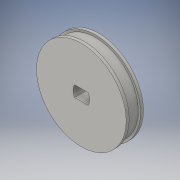
# Autodesk Inventor part: big tire sumo robot
Saved by Autodesk Inventor 2016 (Build 200138000, 138)
## iProperties
Created: 2017-09-06
Part Number: big tire sumo robot
Material: Generic
Document SubType Name: Modeling
Designer: student
Density: 1 g/cm^3
Appearance: Default
Author: student
Autodesk Inventor part; units mm, degrees
ref_plane "YZ Plane" through (0, 0, 0) normal (1, 0, 0) x (0, 1, 0)
ref_plane "XZ Plane" through (0, 0, 0) normal (0, 1, 0) x (-1, 0, 0)
ref_plane "XY Plane" through (0, 0, 0) normal (0, 0, 1) x (1, 0, 0)
sketch "Sketch1" plane through (0, 0, 0) normal (0, 0, 1) x (1, 0, 0)
  circle A0 centre (0, 0) radius 18.1229
  circle A1 centre (0, 0) radius 18.9615
  dimension "d0" = 36.2458
  constraints: 2 centre point, 1 coincident
  measures "d0" diameter of A0
extrude "Extrusion3" add sketch "Sketch1" along normal blind 4.826 contours A0
sketch "Sketch4" plane through (0, 0, 4.826) normal (0, 0, 1) x (1, 0, 0)
  circle A0 centre (0, 0) radius 19.05
  dimension "d17" = 38.1
  constraints: 1 centre point, 1 coincident
  measures "d17" diameter of A0
extrude "Extrusion4" add sketch "Sketch4" along normal blind 1.27
sketch "Sketch5" plane through (0, 0, 0) normal (0, 0, -1) x (-1, 0, 0)
  circle A0 centre (0, 0) radius 19.05
  dimension "d18" = 38.1
  constraints: 1 centre point, 1 coincident
  measures "d18" diameter of A0
extrude "Extrusion5" add sketch "Sketch5" along normal blind 1.27
sketch "Sketch6" plane through (0, 0, 6.096) normal (0, 0, 1) x (1, 0, 0)
  line L0 (2.8729, -2.3622) -> (-2.8729, -2.3622)
  line L1 (2.8729, 2.3622) -> (-2.8729, 2.3622)
  arc A0 (2.8729, -2.3622) -> (2.8729, 2.3622) centre (-1.1303, 0) ccw
  arc A1 (-2.8729, 2.3622) -> (-2.8729, -2.3622) centre (1.1303, 0) ccw
  line L2 (3.5179, 0) -> (-3.5179, 0)
  line L3 (0, 2.3622) -> (0, -2.3622)
  dimension "d23" = 4.7244
  dimension "d24" = 4.6482
  dimension "d25" = 4.6482
  dimension "d26" = 7.0358
  constraints: 8 end point, 6 point on circle, 2 centre point, 2 horizontal, 2 midpoint
  measures "d23" distance between parallel lines of L1 L0
  measures "d24" radius of A0
  measures "d25" radius of A1
extrude "Extrusion7" cut sketch "Sketch6" against normal blind 25.4
body "Solid3"
